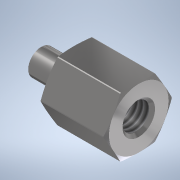
# Autodesk Inventor part: MSU-306-03
Saved by Autodesk Inventor 2020.4 (Build 244396000, 396)
## iProperties
Created: 2016-05-23
Part Number: MSU-306-03
Catalog Web Link: www.cadenas.de
Description: BSLCG, PSLCG, SLCG-Small Hexagonal Posts - One End Male Thread, One End Female Thread Type
Vendor: MISUMI
Document SubType Name: Modeling
Designer: psAdmin
Manufacturer: MISUMI
Mass: 1.16015 g
Surface Area: 2.18726 cm^2
Volume: 0.149697 cm^3
Density: 7.75 g/cm^3
Material: ステンレス鋼 440C
Appearance: 半つや出し
Category: PARTsolutions
Company: MISUMI
PSOL_IDENT_0: {$CADENAS_DATA\23d-libs\misumi\metric\19_posts_stands\pslcg.prj},181 {VTYP=3D},{NB=SLCG5.5-6},{LINA=
PSOL_IDENT_1: SLCG5.5-6},{NN=BSLCG, PSLCG, SLCG},{DATE=08.01.2016 02:52:25},{GEOMDATE=27.05.2011 04:16:00},{VERSIO
PSOL_IDENT_2: N=},{LINEID=30},{LINESUBID=-1},{WBVAR=MAT,ST,LS}  {NB=SLCG5.5-6},{LINA=SLCG5.5-6},{KT=DUMMY},{PN=SLC
PSOL_IDENT_3: G5.5-6},{TYPE=SLCG},{TS=G},{MAT=2},{MATALG= '1', '1018 Carbon Steel', '2', '303 Stainless Steel' },{
PSOL_IDENT_4: ST=},{STALG= '', '-' },{B=5.5},{LS=6},{LSALG=5,6,7,8,9,10,11,12,13,14,15,16,17,18,20},{M=M3},{M1=3.0
PSOL_IDENT_5: 00},{LL=6},{LL1=4},{C=6.3},{MMIN=2.4590},{CON=1}
NN: BSLCG, PSLCG, SLCG
NT: Small Hexagonal Posts - One End Male Thread, One End Female Thread Type
NB: SLCG5.5-6
NBSYN: $PN.
LINA: SLCG5.5-6
PN: SLCG5.5-6
MAT: 303 Stainless Steel
ST: -
B: 5.5
LS: 6
M: M3
LL: 6
LL1: 4
C: 6.3
SUPPLIER: MISUMI
ARTICLENO: SLCG5.5-6
BOMINFO: SLCG5.5-6
CREATOR: CADENAS GmbH
Title: SLCG5.5-6
Author: Cadenas PARTsolutions
Comments: Small Hexagonal Posts - One End Male Thread, One End Female Thread Type
Autodesk Inventor part; units mm, degrees
ref_plane "YZ Plane" through (0, 0, 0) normal (1, 0, 0) x (0, 1, 0)
ref_plane "XZ Plane" through (0, 0, 0) normal (0, 1, 0) x (-1, 0, 0)
ref_plane "XY Plane" through (0, 0, 0) normal (0, 0, 1) x (1, 0, 0)
sketch "Sketch_1" plane through (0, 0, 0) normal (0, 0, 1) x (1, 0, 0)
  line L0 (6, 0) -> (0, 0)
  line L1 (0, 0) -> (0, 2.75)
  line L2 (0, 2.75) -> (0.1072, 3.15)
  line L3 (0.1072, 3.15) -> (5.8928, 3.15)
  line L4 (5.8928, 3.15) -> (6, 2.75)
  line L5 (6, 2.75) -> (6, 0)
  line L6 (6, 0) -> (0, 0)
  constraints: 14 end point
revolve "Revolution1" add sketch "Sketch_1" angle 360 about axis through (6, 0, 0) along (1, 0, 0)
sketch "Sketch_5" plane through (0, 0, 0) normal (0, 0, 1) x (1, 0, 0)
  line L0 (0, 0) -> (-6, 0)
  line L1 (-6, 0) -> (-6, 1.1935)
  line L2 (-6, 1.1935) -> (-5.6935, 1.5)
  line L3 (-5.6935, 1.5) -> (-0.6, 1.5)
  line L4 (-0.6, 1.5) -> (-0.6, 1.2295)
  line L5 (-0.6, 1.2295) -> (0, 1.2295)
  line L6 (0, 1.2295) -> (0, 0)
  line L7 (0, 0) -> (-6, 0)
  constraints: 16 end point
revolve "Revolution2" add sketch "Sketch_5" angle 360 about axis through (0, 0, 0) along (1, 0, 0)
thread "Thread1" size "M3x0.5" class "6g" standard "ISO Metric profile" full length
sketch "Sketch_6" plane through (0, 0, 0) normal (1, 0, 0) x (0, 1, 0)
  circle A0 centre (0, 0) radius 6.3
  line L0 (1.5877, 2.75) -> (-1.5877, 2.75)
  line L1 (-1.5877, 2.75) -> (-3.1754, 0)
  line L2 (-3.1754, 0) -> (-1.5877, -2.75)
  line L3 (-1.5877, -2.75) -> (1.5877, -2.75)
  line L4 (1.5877, -2.75) -> (3.1754, 0)
  line L5 (3.1754, 0) -> (1.5877, 2.75)
  constraints: 12 end point, 1 centre point
extrude "Extrusion1" cut sketch "Sketch_6" along normal blind 6
sketch "Sketch4" plane through (6, 0, 0) normal (1, 0, 0) x (0, 0, -1)
  point P0 (0, 0)
hole "Hole1" at (6, 0, 0) direction (-1, 0, 0) diameter 2.459 depth 4.0901 tip angle 120 countersink diameter 3 countersink angle 90 thread size "M3x0.5" class "6H" standard "ISO Metric profile"
sketch "スケッチ5" plane through (-6, 0, 0) normal (-1, 0, 0) x (0, 0, 1)
  circle A0 centre (0, 0) radius 1.1935 projected
  circle A1 centre (0, 0) radius 1.2
  circle A2 centre (0, 0) radius 2.1125
  dimension "d13" = 2.4
  constraints: 2 centre point, 2 coincident
  measures "d13" diameter of A1
extrude "押し出し2" cut sketch "スケッチ5" against normal blind 6 contours A2
sketch "スケッチ6" plane through (-6, 0, 0) normal (-1, 0, 0) x (0, 0, 1)
  circle A0 centre (0, 0) radius 1.1935 projected
  circle A1 centre (0, 0) radius 4.3291
  constraints: 1 centre point, 1 coincident
extrude "押し出し3" cut sketch "スケッチ6" against normal blind 3 contours A0 | A1
sketch "スケッチ7" plane through (0, 0, 0) normal (0, 1, 0) x (-1, 0, 0)
  line L0 (0, 1.375) -> (0, -1.375) projected
  line L1 (10.0538, 0) -> (-16.076, 0)
  line L2 (-0.1072, 0.0446) -> (-0.1072, -0.0446) projected
  line L3 (10.0538, 0) -> (7.865, -1.944)
  line L4 (10.0538, 0) -> (7.865, 1.944)
  line L5 (-16.076, 0) -> (-13.8872, -1.944)
  line L6 (-16.076, 0) -> (-13.8872, 1.944)
  point P0 (0, 0)
  point P1 (0, 0)
  point P2 (-0.1072, 0)
  constraints: 10 end point, 2 midpoint, 2 symmetric about line, 1 equal length, 1 horizontal, 1 horizontal alignment, 1 point on line
body "Solid1"
